Autodesk Inventor part; units mm, degrees
(part 2 of 2)
sketch "Sketch13" plane through (-19.0722, 68, 73.5) normal (0, 1, 0) x (1, 0, 0)
  line L0 (-55.4278, 71.5) -> (-52.4278, 71.5) projected
  line L1 (-55.4278, 75.5) -> (-55.4278, 71.5) projected
  line L2 (-52.4278, 75.5) -> (-55.4278, 75.5) projected
  line L3 (-52.4278, 71.5) -> (-52.4278, 75.5) projected
  line L4 (19.0722, 73.5) -> (-52.4278, 73.5)
  line L5 (-52.4278, 75.5) -> (-52.4278, 71.5)
  line L6 (-55.4278, 71.5) -> (-55.4278, 75.5)
  line L7 (-55.4278, 75.5) -> (-52.4278, 75.5)
  line L8 (-55.4278, 71.5) -> (-52.4278, 71.5)
  arc A0 (-0.5155, 146.9324) -> (-0.5155, 0.0676) centre (19.0722, 73.5) ccw projected
  arc A1 (27.1963, 76) -> (27.1963, 71) centre (19.0722, 73.5) ccw projected
  circle A2 centre (19.0722, 73.5) radius 76
  line L9 (-53.7416, 57.6129) -> (-50.8287, 58.3308)
  line L10 (-52.7843, 53.7291) -> (-53.7416, 57.6129)
  line L11 (-52.7843, 53.7291) -> (-49.8715, 54.447)
  line L12 (-50.8287, 58.3308) -> (-49.8715, 54.447)
  line L13 (-47.8237, 40.649) -> (-45.1673, 42.0432)
  line L14 (-45.9648, 37.1072) -> (-47.8237, 40.649)
  line L15 (-45.9648, 37.1072) -> (-43.3084, 38.5014)
  line L16 (-45.1673, 42.0432) -> (-43.3084, 38.5014)
  line L17 (-38.0181, 25.5944) -> (-35.7725, 27.5838)
  line L18 (-35.3656, 22.6003) -> (-38.0181, 25.5944)
  line L19 (-35.3656, 22.6003) -> (-33.12, 24.5897)
  line L20 (-35.7725, 27.5838) -> (-33.12, 24.5897)
  line L21 (-24.8946, 13.3238) -> (-23.1904, 15.7928)
  line L22 (-21.6026, 11.0516) -> (-24.8946, 13.3238)
  line L23 (-21.6026, 11.0516) -> (-19.8984, 13.5205)
  line L24 (-23.1904, 15.7928) -> (-19.8984, 13.5205)
  line L25 (-9.2159, 4.5505) -> (-8.1521, 7.3555)
  line L26 (-5.4758, 3.1321) -> (-9.2159, 4.5505)
  line L27 (-5.4758, 3.1321) -> (-4.412, 5.9371)
  line L28 (-8.1521, 7.3555) -> (-4.412, 5.9371)
  line L29 (8.1068, -0.2157) -> (8.4684, 2.7624)
  line L30 (12.0777, -0.6979) -> (8.1068, -0.2157)
  line L31 (12.0777, -0.6979) -> (12.4393, 2.2802)
  line L32 (8.4684, 2.7624) -> (12.4393, 2.2802)
  line L33 (26.0668, -0.6979) -> (25.7052, 2.2802)
  line L34 (30.0376, -0.2157) -> (26.0668, -0.6979)
  line L35 (30.0376, -0.2157) -> (29.676, 2.7624)
  line L36 (25.7052, 2.2802) -> (29.676, 2.7624)
  line L37 (43.6203, 3.1321) -> (42.5564, 5.9371)
  line L38 (47.3603, 4.5505) -> (43.6203, 3.1321)
  line L39 (47.3603, 4.5505) -> (46.2965, 7.3555)
  line L40 (42.5564, 5.9371) -> (46.2965, 7.3555)
  line L41 (59.7471, 11.0516) -> (58.0429, 13.5205)
  line L42 (63.039, 13.3238) -> (59.7471, 11.0516)
  line L43 (63.039, 13.3238) -> (61.3348, 15.7928)
  line L44 (58.0429, 13.5205) -> (61.3348, 15.7928)
  line L45 (73.51, 22.6003) -> (71.2645, 24.5897)
  line L46 (76.1625, 25.5944) -> (73.51, 22.6003)
  line L47 (76.1625, 25.5944) -> (73.917, 27.5838)
  line L48 (71.2645, 24.5897) -> (73.917, 27.5838)
  line L49 (84.1093, 37.1072) -> (81.4529, 38.5014)
  line L50 (85.9682, 40.649) -> (84.1093, 37.1072)
  line L51 (85.9682, 40.649) -> (83.3118, 42.0432)
  line L52 (81.4529, 38.5014) -> (83.3118, 42.0432)
  line L53 (90.9288, 53.7291) -> (88.0159, 54.447)
  line L54 (91.886, 57.6129) -> (90.9288, 53.7291)
  line L55 (91.886, 57.6129) -> (88.9732, 58.3308)
  line L56 (88.0159, 54.447) -> (88.9732, 58.3308)
  line L57 (93.5722, 71.5) -> (90.5722, 71.5)
  line L58 (93.5722, 75.5) -> (93.5722, 71.5)
  line L59 (93.5722, 75.5) -> (90.5722, 75.5)
  line L60 (90.5722, 71.5) -> (90.5722, 75.5)
  line L61 (91.886, 89.3871) -> (88.9732, 88.6692)
  line L62 (90.9288, 93.2709) -> (91.886, 89.3871)
  line L63 (90.9288, 93.2709) -> (88.0159, 92.553)
  line L64 (88.9732, 88.6692) -> (88.0159, 92.553)
  line L65 (85.9682, 106.351) -> (83.3118, 104.9568)
  line L66 (84.1093, 109.8928) -> (85.9682, 106.351)
  line L67 (84.1093, 109.8928) -> (81.4529, 108.4986)
  line L68 (83.3118, 104.9568) -> (81.4529, 108.4986)
  line L69 (76.1625, 121.4056) -> (73.917, 119.4162)
  line L70 (73.51, 124.3997) -> (76.1625, 121.4056)
  line L71 (73.51, 124.3997) -> (71.2645, 122.4103)
  line L72 (73.917, 119.4162) -> (71.2645, 122.4103)
  line L73 (63.039, 133.6762) -> (61.3348, 131.2072)
  line L74 (59.7471, 135.9484) -> (63.039, 133.6762)
  line L75 (59.7471, 135.9484) -> (58.0429, 133.4795)
  line L76 (61.3348, 131.2072) -> (58.0429, 133.4795)
  line L77 (47.3603, 142.4495) -> (46.2965, 139.6445)
  line L78 (43.6203, 143.8679) -> (47.3603, 142.4495)
  line L79 (43.6203, 143.8679) -> (42.5564, 141.0629)
  line L80 (46.2965, 139.6445) -> (42.5564, 141.0629)
  line L81 (30.0376, 147.2157) -> (29.676, 144.2376)
  line L82 (26.0668, 147.6979) -> (30.0376, 147.2157)
  line L83 (26.0668, 147.6979) -> (25.7052, 144.7198)
  line L84 (29.676, 144.2376) -> (25.7052, 144.7198)
  line L85 (12.0777, 147.6979) -> (12.4393, 144.7198)
  line L86 (8.1068, 147.2157) -> (12.0777, 147.6979)
  line L87 (8.1068, 147.2157) -> (8.4684, 144.2376)
  line L88 (12.4393, 144.7198) -> (8.4684, 144.2376)
  line L89 (-5.4758, 143.8679) -> (-4.412, 141.0629)
  line L90 (-9.2159, 142.4495) -> (-5.4758, 143.8679)
  line L91 (-9.2159, 142.4495) -> (-8.1521, 139.6445)
  line L92 (-4.412, 141.0629) -> (-8.1521, 139.6445)
  line L93 (-21.6026, 135.9484) -> (-19.8984, 133.4795)
  line L94 (-24.8946, 133.6762) -> (-21.6026, 135.9484)
  line L95 (-24.8946, 133.6762) -> (-23.1904, 131.2072)
  line L96 (-19.8984, 133.4795) -> (-23.1904, 131.2072)
  line L97 (-35.3656, 124.3997) -> (-33.12, 122.4103)
  line L98 (-38.0181, 121.4056) -> (-35.3656, 124.3997)
  line L99 (-38.0181, 121.4056) -> (-35.7725, 119.4162)
  line L100 (-33.12, 122.4103) -> (-35.7725, 119.4162)
  line L101 (-45.9648, 109.8928) -> (-43.3084, 108.4986)
  line L102 (-47.8237, 106.351) -> (-45.9648, 109.8928)
  line L103 (-47.8237, 106.351) -> (-45.1673, 104.9568)
  line L104 (-43.3084, 108.4986) -> (-45.1673, 104.9568)
  line L105 (-52.7843, 93.2709) -> (-49.8715, 92.553)
  line L106 (-53.7416, 89.3871) -> (-52.7843, 93.2709)
  line L107 (-53.7416, 89.3871) -> (-50.8287, 88.6692)
  line L108 (-49.8715, 92.553) -> (-50.8287, 88.6692)
  line L109 (26.4753, 1.6868) -> (30.4753, 1.6868) projected
  line L110 (26.4753, 4.3868) -> (26.4753, 1.6868) projected
  line L111 (30.4753, 4.3868) -> (26.4753, 4.3868) projected
  line L112 (30.4753, 1.6868) -> (30.4753, 4.3868) projected
  line L113 (11.6692, 4.3868) -> (7.6692, 4.3868) projected
  line L114 (7.6692, 4.3868) -> (7.6692, 1.6868) projected
  line L115 (7.6692, 1.6868) -> (11.6692, 1.6868) projected
  line L116 (11.6692, 1.6868) -> (11.6692, 4.3868) projected
  line L117 (11.6692, 145.3132) -> (7.6692, 145.3132) projected
  line L118 (7.6692, 145.3132) -> (7.6692, 142.6132) projected
  line L119 (7.6692, 142.6132) -> (11.6692, 142.6132) projected
  line L120 (11.6692, 142.6132) -> (11.6692, 145.3132) projected
  line L121 (26.4753, 145.3132) -> (26.4753, 142.6132) projected
  line L122 (26.4753, 142.6132) -> (30.4753, 142.6132) projected
  line L123 (30.4753, 142.6132) -> (30.4753, 145.3132) projected
  line L124 (30.4753, 145.3132) -> (26.4753, 145.3132) projected
  line L125 (65.7222, 108.0505) -> (68.4222, 108.0505) projected
  line L126 (65.7222, 112.0505) -> (65.7222, 108.0505) projected
  line L127 (68.4222, 108.0505) -> (68.4222, 112.0505) projected
  line L128 (68.4222, 112.0505) -> (65.7222, 112.0505) projected
  line L129 (65.7222, 87.6835) -> (65.7222, 83.6835) projected
  line L130 (65.7222, 83.6835) -> (68.4222, 83.6835) projected
  line L131 (68.4222, 83.6835) -> (68.4222, 87.6835) projected
  line L132 (68.4222, 87.6835) -> (65.7222, 87.6835) projected
  line L133 (68.4222, 63.3165) -> (65.7222, 63.3165) projected
  line L134 (65.7222, 63.3165) -> (65.7222, 59.3165) projected
  line L135 (65.7222, 59.3165) -> (68.4222, 59.3165) projected
  line L136 (68.4222, 59.3165) -> (68.4222, 63.3165) projected
  line L137 (68.4222, 38.9495) -> (65.7222, 38.9495) projected
  line L138 (65.7222, 38.9495) -> (65.7222, 34.9495) projected
  line L139 (68.4222, 34.9495) -> (68.4222, 38.9495) projected
  line L140 (65.7222, 34.9495) -> (68.4222, 34.9495) projected
  point P0 (11.6692, 144.6262)
  point P1 (8.3378, 145.3132)
  dimension "d177" = 152
  dimension "d180" = 360
  constraints: 210 end point, 4 collinear, 1 centre point, 1 coincident, 1 concentric, 1 midpoint, 209 other
  measures "d177" diameter of A2
extrude "Extrusion11" cut sketch "Sketch13" against normal blind 3 contours L1 L2 L3 L0 | L9 L12 L11 L10 | L13 L16 L15 L14 | L17 L20 L19 L18 | L21 L24 L23 L22 | L25 L28 L27 L26 | L115 L114 L113 L116 L32 L29 | L29 L32 L116 L115 | L110 L111 L112 L109 L35 L36 | L36 L35 L109 L110 | L37 L40 L39 L38 | L41 L44 L43 L42 | L73 L76 L75 L74 | L77 L80 L79 L78 | L124 L123 L122 L121 L84 L81 | L81 L84 L121 L124 | L120 L119 L118 L117 L87 L88 | L88 L87 L117 L120 | L89 L92 L91 L90 | L93 L96 L95 L94 | L97 L100 L99 L98 | L101 L104 L103 L102 | L105 L108 L107 L106 | L126 L128 L127 L125 | L132 L131 L130 L129 | L136 L135 L134 L133 | L139 L140 L138 L137 bodies 2
body "Solid1"
body "Solid2"
body "Solid3"
